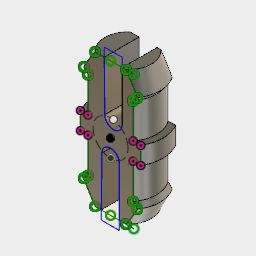
stuby v2 (Autodesk Fusion 360 design; units mm, degrees)
Autodesk Fusion 360 part; units mm, degrees
note: some values were not read from the file. Set by a fixed rule: which sketch regions a step uses.
sketch "Sketch1" plane through (0, 0, 0) normal (0, 1, 0) x (1, 0, 0)
  line L0 (3, 0) -> (3, -0.75)
  line L1 (3, -0.75) -> (2.45, -0.75)
  line L2 (2.45, -0.75) -> (2.45, -3.75)
  line L3 (2.45, -3.75) -> (2.75, -4.1489)
  line L4 (2.75, -4.1489) -> (2, -5.75)
  line L5 (2, -5.75) -> (0, -5.75)
  line L6 (3, 0) -> (0, 0) construction
  line L7 (2.75, 4.1489) -> (2, 5.75)
  line L8 (3, 0) -> (3, 0.75)
  line L9 (2.45, 0.75) -> (2.45, 3.75)
  line L10 (2.45, 3.75) -> (2.75, 4.1489)
  line L11 (2, 5.75) -> (0, 5.75)
  line L12 (0, 0) -> (0, 6.5) construction
  line L13 (3, 0.75) -> (2.45, 0.75)
  line L14 (0, -5.75) -> (0, 5.75)
  dimension "d1" = 3
  dimension "d2" = 0.75
  dimension "d3" = 3
  dimension "d4" = 5
  dimension "d6" = 2
  dimension "d7" = 2.75
  dimension "d8" = 2.45
  dimension "d9" = 2
  measures "d1" distance of L6.end L0.start
  measures "d2" distance of L0.start L0.end
  measures "d3" distance of L1.end L2.end
  measures "d4" distance of L1 L5
  measures "d6" distance of L6.end L4.end
  measures "d7" distance of L6.end L3.end
  measures "d8" distance of L6.end L2
  measures "d9" distance of L4.end L5.end
revolve "Revolve2" add sketch "Sketch1" angle 360 about axis through (0, 0, 5.75) along (0, 0, -1)
sketch "Sketch3" plane through (0, 0, 5.75) normal (0, 0, 1) x (-1, 0, 0)
  circle A0 centre (0, 0) radius 2
  line L0 (-5, -1.5) -> (5, -1.5)
  line L1 (5, -1.5) -> (5, 1.5)
  line L2 (5, 1.5) -> (-5, 1.5)
  line L3 (-5, 1.5) -> (-5, -1.5)
  line L4 (-5, -1.5) -> (5, 1.5) construction
  line L5 (5, -1.5) -> (-5, 1.5) construction
  line L6 (5.6117, 3.0022) -> (-6, 3.0022)
  line L7 (-6, 3.0022) -> (-6, -3)
  line L8 (-6, -3) -> (5.6117, -3)
  line L9 (5.6117, -3) -> (5.6117, 3.0022)
  circle A1 centre (0, 0) radius 2
  dimension "d12" = 10
  dimension "d13" = 3
  measures "d12" distance of L1.end L2.end
  measures "d13" distance of L0.end L1.end
extrude "Extrude3" cut sketch "Sketch3" against normal blind 14 contours A0 L2 A1 | A0 L0 A1 | L6 L7 L8 L9
sketch "Sketch4" plane through (0, -1.5, 0) normal (0, -1, 0) x (1, 0, 0)
  spline S0 degree 2 poles (-2.3049, 4.1489) (-1.7364, 5.1662) (-1.3229, 5.75) knots 0 0 0 0.187886 0.187886 0.187886 weights 1 1.022081 1
  spline S1 degree 2 poles (-1.9371, 3.75) (-2.1104, 3.9322) (-2.3049, 4.1489) knots 0 0 0 0.054258 0.054258 0.054258 weights 1 1.00251 1
  line L0 (-1.9371, 3.75) -> (-1.9371, 0.75)
  line L1 (-1.9371, 0.75) -> (-2.5981, 0.75)
  line L2 (-2.5981, 0.75) -> (-2.5981, -0.75)
  line L3 (-2.5981, -0.75) -> (-1.9371, -0.75)
  line L4 (-1.9371, -0.75) -> (-1.9371, -3.75)
  spline S2 degree 2 poles (-2.3049, -4.1489) (-2.1104, -3.9322) (-1.9371, -3.75) knots 0 0 0 0.054258 0.054258 0.054258 weights 1 1.00251 1
  spline S3 degree 2 poles (-1.3229, -5.75) (-1.7364, -5.1662) (-2.3049, -4.1489) knots 0 0 0 0.187886 0.187886 0.187886 weights 1 1.022081 1
  line L5 (-1.3229, -5.75) -> (1.3229, -5.75)
  spline S4 degree 2 poles (2.3049, -4.1489) (1.7364, -5.1662) (1.3229, -5.75) knots 0 0 0 0.187886 0.187886 0.187886 weights 1 1.022081 1
  spline S5 degree 2 poles (1.9371, -3.75) (2.1104, -3.9322) (2.3049, -4.1489) knots 0 0 0 0.054258 0.054258 0.054258 weights 1 1.00251 1
  line L6 (1.9371, -3.75) -> (1.9371, -0.75)
  line L7 (1.9371, -0.75) -> (2.5981, -0.75)
  line L8 (2.5981, -0.75) -> (2.5981, 0.75)
  line L9 (2.5981, 0.75) -> (1.9371, 0.75)
  line L10 (1.9371, 0.75) -> (1.9371, 3.75)
  spline S6 degree 2 poles (2.3049, 4.1489) (2.1104, 3.9322) (1.9371, 3.75) knots 0 0 0 0.054258 0.054258 0.054258 weights 1 1.00251 1
  spline S7 degree 2 poles (1.3229, 5.75) (1.7364, 5.1662) (2.3049, 4.1489) knots 0 0 0 0.187886 0.187886 0.187886 weights 1 1.022081 1
  line L11 (1.3229, 5.75) -> (-1.3229, 5.75)
  circle A0 centre (0, 0) radius 1.5 construction
  line L12 (-0.5432, 5.75) -> (-0.5, 1.4958)
  line L13 (2, 5.75) -> (0, 5.75)
  line L14 (1, 5.75) -> (1, 1.5034)
  line L15 (2, -5.75) -> (0, -5.75)
  line L16 (-0.75, -1.4919) -> (-0.7961, -5.75)
  arc A1 (0.7487, -1.4562) -> (-0.75, -1.4919) centre (0, -1.5) ccw
  line L17 (-0.7961, -5.75) -> (-0.7961, -6.4979)
  line L18 (-0.7961, -6.4979) -> (0.7464, -6.5067)
  line L19 (-0.5432, 5.75) -> (-0.5402, 6.4921)
  line L20 (-0.5402, 6.4921) -> (1, 6.5078)
  line L21 (1, 5.75) -> (1, 6.5078)
  arc A2 (-0.5, 1.4958) -> (1, 1.5034) centre (0.25, 1.5034) ccw
  spline S8 degree 2 poles (-2.3049, 4.1489) (-1.7364, 5.1662) (-1.3229, 5.75) knots 0 0 0 0.187886 0.187886 0.187886 weights 1 1.022081 1
  spline S9 degree 2 poles (-1.9371, 3.75) (-2.1104, 3.9322) (-2.3049, 4.1489) knots 0 0 0 0.054258 0.054258 0.054258 weights 1 1.00251 1
  line L22 (-1.9371, 3.75) -> (-1.9371, 0.75)
  line L23 (-1.9371, 0.75) -> (-2.5981, 0.75)
  line L24 (-2.5981, 0.75) -> (-2.5981, -0.75)
  line L25 (-2.5981, -0.75) -> (-1.9371, -0.75)
  line L26 (-1.9371, -0.75) -> (-1.9371, -3.75)
  spline S10 degree 2 poles (-2.3049, -4.1489) (-2.1104, -3.9322) (-1.9371, -3.75) knots 0 0 0 0.054258 0.054258 0.054258 weights 1 1.00251 1
  spline S11 degree 2 poles (-1.3229, -5.75) (-1.7364, -5.1662) (-2.3049, -4.1489) knots 0 0 0 0.187886 0.187886 0.187886 weights 1 1.022081 1
  line L27 (-1.3229, -5.75) -> (1.3229, -5.75)
  spline S12 degree 2 poles (2.3049, -4.1489) (1.7364, -5.1662) (1.3229, -5.75) knots 0 0 0 0.187886 0.187886 0.187886 weights 1 1.022081 1
  spline S13 degree 2 poles (1.9371, -3.75) (2.1104, -3.9322) (2.3049, -4.1489) knots 0 0 0 0.054258 0.054258 0.054258 weights 1 1.00251 1
  line L28 (1.9371, -3.75) -> (1.9371, -0.75)
  line L29 (1.9371, -0.75) -> (2.5981, -0.75)
  line L30 (2.5981, -0.75) -> (2.5981, 0.75)
  line L31 (2.5981, 0.75) -> (1.9371, 0.75)
  line L32 (1.9371, 0.75) -> (1.9371, 3.75)
  spline S14 degree 2 poles (2.3049, 4.1489) (2.1104, 3.9322) (1.9371, 3.75) knots 0 0 0 0.054258 0.054258 0.054258 weights 1 1.00251 1
  spline S15 degree 2 poles (1.3229, 5.75) (1.7364, 5.1662) (2.3049, 4.1489) knots 0 0 0 0.187886 0.187886 0.187886 weights 1 1.022081 1
  line L33 (1.3229, 5.75) -> (-1.3229, 5.75)
  line L34 (0.7487, -1.4562) -> (0.7464, -6.5067)
  dimension "d16" = 3
  dimension "d17" = 1.5
  dimension "d18" = 1.5
  measures "d16" diameter of A0
  measures "d17" diameter of A2
  measures "d18" diameter of A1
extrude "Extrude4" cut sketch "Sketch4" against normal blind 6 contours L11 L13 L19 L20 L21 L33 | L11 L12 L13 L14 A2 L33 | L5 L15 L16 A1 L27 L34 | L5 L15 L17 L18 L27 L34
equation "d2 = 0.8 mm - 0.05 mm"
